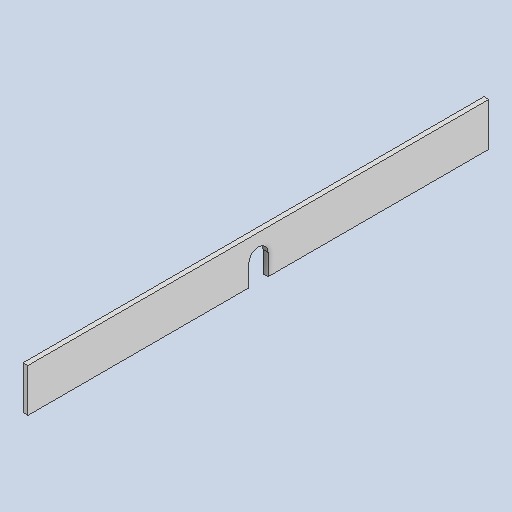
# Autodesk Inventor part: PlateExt
Saved by Autodesk Inventor 2023 (Build 270158030, 158C)
## iProperties
Created: 2022-07-27
Part Number: PlateExt
Material: Generic
Document SubType Name: Modeling
Designer: jeremyy
Density: 1 g/cm^3
Appearance: Default
Author: jeremyy
Autodesk Inventor part; units mm, degrees
ref_plane "YZ Plane" through (0, 0, 0) normal (1, 0, 0) x (0, 1, 0)
ref_plane "XZ Plane" through (0, 0, 0) normal (0, 1, 0) x (-1, 0, 0)
ref_plane "XY Plane" through (0, 0, 0) normal (0, 0, 1) x (1, 0, 0)
sketch "Sketch1" plane through (0, 0, 0) normal (1, 0, 0) x (0, 1, 0)
  line L0 (0, 0) -> (0, -304.8)
  line L1 (0, -304.8) -> (28.575, -304.8)
  line L2 (28.575, -304.8) -> (28.575, 0)
  line L3 (28.575, 0) -> (0, 0)
  line L4 (0, -146.05) -> (13.97, -146.05)
  line L5 (0, -158.75) -> (13.97, -158.75)
  arc A0 (13.97, -158.75) -> (13.97, -146.05) centre (13.97, -152.4) ccw
  point P0 (20.32, -152.4)
  dimension "d0" = 304.8
  dimension "d1" = 28.575
  dimension "d2" = 146.05
  dimension "d3" = 146.05
  dimension "d5" = 20.32
  constraints: 12 end point, 3 perpendicular, 3 point on circle, 2 point on line, 1 centre point, 1 horizontal, 1 parallel, 1 tangent, 1 vertical
  measures "d0" distance of L0.start L0.end
  measures "d1" distance of L0.end L1.end
  measures "d2" distance of L0.start L4.start
  measures "d3" distance of L0.end L5.start
  measures "d5" distance from line of L0 point (20.32, -152.4)
extrude "Extrusion1" add sketch "Sketch1" along normal blind 3.175 contours L3 L2 L1 L0 L5 A0 L4
body "Solid1"
